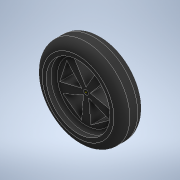
# Autodesk Inventor part: Wheel 2
Saved by Autodesk Inventor 2021 (Build 250183000, 183)
## iProperties
Created: 2021-06-29
Part Number: Wheel 2
Material: Rubber
Document SubType Name: Modeling
Designer: Manojgouda K R
Density: 0.93 g/cm^3
Appearance: Rubber - Black
Author: Manojgouda K R
Autodesk Inventor part; units mm, degrees
ref_plane "YZ Plane" through (0, 0, 0) normal (1, 0, 0) x (0, 1, 0)
ref_plane "XZ Plane" through (0, 0, 0) normal (0, 1, 0) x (-1, 0, 0)
ref_plane "XY Plane" through (0, 0, 0) normal (0, 0, 1) x (1, 0, 0)
sketch "Sketch1" plane through (0, 0, 0) normal (0, 0, 1) x (1, 0, 0)
  circle A0 centre (0, 0) radius 2.75
  circle A1 centre (0, 0) radius 2
  dimension "d0" = 5.5
  dimension "d1" = 4
  constraints: 2 centre point, 2 coincident
  measures "d0" diameter of A0
  measures "d1" diameter of A1
extrude "Extrusion1" add sketch "Sketch1" along normal blind 1.5 contours A0 | A1
sketch "Sketch2" plane through (0, 0, 1.5) normal (0, 0, 1) x (1, 0, 0)
  circle A0 centre (0, 0) radius 2
  dimension "d4" = 4
  constraints: 1 centre point, 1 coincident
  measures "d4" diameter of A0
extrude "Extrusion2" cut sketch "Sketch2" against normal blind 0.5
fillet "Fillet1" radius 0.5 2 edges at (-2.75, 0, 1.5) (-2.75, 0, 0)
fillet "Fillet2" radius 0.2 1 edges at (-2, 0, 1)
sketch "Sketch3" plane through (0, 0, 1) normal (0, 0, 1) x (1, 0, 0)
  point P0 (0, 0)
sketch "Sketch4" plane through (0, 0, 1) normal (0, 0, 1) x (1, 0, 0)
  line L0 (-0.749, 1.5) -> (0, 0.278)
  line L1 (0, 0.278) -> (0.7058, 1.5)
  line L2 (0.7058, 1.5) -> (-0.749, 1.5)
  circle A0 centre (0, 0) radius 2 projected
  dimension "d9" = 0.5
  constraints: 6 end point, 1 horizontal
  measures "d9" distance edge to line of A0 L2
extrude "Extrusion3" cut sketch "Sketch4" against normal through all contours L2 L1 L0
pattern_circular "Circular Pattern1" count 5 over 360 about axis through (0, 0, 1.2) along (0, 0, -1) of "Extrusion3"
sketch "Sketch5" plane through (0, 0, 1) normal (0, 0, 1) x (1, 0, 0)
  circle A0 centre (0, 0) radius 0.15
  dimension "d15" = 0.3
  constraints: 1 centre point, 1 coincident
  measures "d15" diameter of A0
extrude "Extrusion4" cut sketch "Sketch5" against normal through all
body "Solid1"
